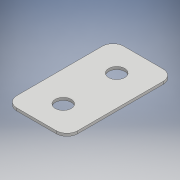
# Autodesk Inventor part: FlexHinge
Saved by Autodesk Inventor 2018 (Build 220112000, 112)
## iProperties
Created: 2018-01-14
Part Number: FlexHinge
Material: Generic
Document SubType Name: Modeling
Designer: reide
Density: 1 g/cm^3
Appearance: Default
Author: reide
Autodesk Inventor part; units mm, degrees
ref_plane "YZ Plane" through (0, 0, 0) normal (1, 0, 0) x (0, 1, 0)
ref_plane "XZ Plane" through (0, 0, 0) normal (0, 1, 0) x (-1, 0, 0)
ref_plane "XY Plane" through (0, 0, 0) normal (0, 0, 1) x (1, 0, 0)
sketch "Sketch1" plane through (0, 0, 0) normal (0, 0, 1) x (1, 0, 0)
  line L0 (55.125, -6.9417) -> (55.125, -0.9417) projected
  line L1 (55.125, -6.9417) -> (66.5, -6.9417) projected
  line L2 (66.5, 3.0583) -> (66.5, -6.9417) projected
  line L3 (66.5, 3.0583) -> (-66.5, 3.0583) projected
  line L4 (-66.5, -6.9417) -> (-66.5, 3.0583) projected
  line L5 (-66.5, -6.9417) -> (-55.125, -6.9417) projected
  line L6 (-55.125, -0.9417) -> (-55.125, -6.9417) projected
  line L7 (55.125, -0.9417) -> (-55.125, -0.9417) projected
  line L8 (-55.125, -6.9417) -> (-55.125, -35.9417) projected
  line L9 (-55.125, -6.9417) -> (-66.5, -6.9417) projected
  line L10 (-66.5, -40.9417) -> (-66.5, -6.9417) projected
  line L11 (-37.5645, -40.9417) -> (-66.5, -40.9417) projected
  line L12 (-37.5645, -38.4017) -> (-37.5645, -40.9417) projected
  line L13 (-37.5645, -38.4017) -> (-28.75, -38.4017) projected
  line L14 (55.125, -35.9417) -> (55.125, -6.9417) projected
  line L15 (28.75, -38.4017) -> (37.5645, -38.4017) projected
  line L16 (37.5645, -40.9417) -> (37.5645, -38.4017) projected
  line L17 (66.5, -40.9417) -> (37.5645, -40.9417) projected
  line L18 (66.5, -6.9417) -> (66.5, -40.9417) projected
  line L19 (55.125, -6.9417) -> (66.5, -6.9417) projected
  line L20 (-66.5, 3.0583) -> (-55.125, 3.0583)
  line L21 (-55.125, 3.0583) -> (-55.125, -16.9417)
  line L22 (-55.125, -16.9417) -> (-66.5, -16.9417)
  line L23 (-66.5, -16.9417) -> (-66.5, 3.0583)
  line L24 (-66.5, -6.9417) -> (-66.5, -11.9417)
  circle A0 centre (-60.8125, -1.9417) radius 1.5
  circle A1 centre (-60.8125, -11.9417) radius 1.5
  circle A2 centre (-60.8125, -11.9417) radius 1.375 projected
  circle A3 centre (60.8125, -11.9417) radius 1.375 projected
  circle A4 centre (-60.8125, -1.9417) radius 1.375 projected
  circle A5 centre (60.8125, -1.9417) radius 1.375 projected
  line L25 (-53.125, -37.9417) -> (-28.75, -37.9417) projected
  arc A6 (-55.125, -35.9417) -> (-53.125, -37.9417) centre (-53.125, -35.9417) ccw projected
  line L26 (-28.75, -37.9417) -> (-28.75, -38.4017) projected
  line L27 (28.75, -37.9417) -> (53.125, -37.9417) projected
  line L28 (28.75, -38.4017) -> (28.75, -37.9417) projected
  arc A7 (53.125, -37.9417) -> (55.125, -35.9417) centre (53.125, -35.9417) ccw projected
  point P0 (0, 0)
  point P1 (-60.8125, 3.0583)
  point P2 (-66.5, -1.9417)
  dimension "d0" = 20
  dimension "d1" = 5
  dimension "d2" = 3
  dimension "d4" = 3
  constraints: 10 end point, 3 point on line, 2 centre point, 2 parallel, 1 horizontal, 1 midpoint, 1 perpendicular
  measures "d0" distance between parallel lines of L22 L3
  measures "d1" distance of L4.start L24.end
  measures "d2" diameter of A0
  measures "d4" diameter of A1
extrude "Extrusion1" add sketch "Sketch1" along normal blind 0.5 contours L6 L5 L4 L3 L21 | L8 L22 L10 L5
fillet "Fillet1" radius 2 4 edges at (-66.5, 3.0583, 0.25) (-55.125, 3.0583, 0.25) (-55.125, -16.9417, 0.25) (-66.5, -16.9417, 0.25)
body "Solid1"
